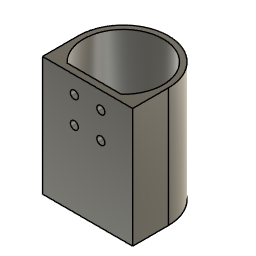
Tube v4 (Autodesk Fusion 360 design; units mm, degrees)
Autodesk Fusion 360 part; units mm, degrees
note: some values were not read from the file. Set by a fixed rule: which sketch regions a step uses.
sketch "Sketch1" plane through (0, 0, 0) normal (0, 0, 1) x (1, 0, 0)
  circle A0 centre (0, 0) radius 30
  circle A1 centre (0, 0) radius 34
  line L0 (0, 30) -> (0, -22) construction
  line L1 (-20.3961, -22) -> (20.3961, -22)
  line L2 (-34, -27) -> (34, -27)
  line L3 (-34, -27) -> (-34, 0)
  line L4 (34, -27) -> (34, 0)
  circle A2 centre (0, 4) radius 25.4 construction
  dimension "d1" = 60
  dimension "d2" = 68
  dimension "d3" = 52
  dimension "d6" = 5
  dimension "d38" = 50.8
  constraint coincident A0.centre A1.centre
  constraint coincident A0 L0.start
  constraint vertical L0
  constraint coincident A0.centre L0
  constraint coincident A0 L1.start
  constraint coincident A0 L1.end
  constraint horizontal L1
  constraint coincident L0.end L1
  constraint parallel L1 L2
  constraint coincident A1 L3.end
  constraint tangent A1 L3
  constraint coincident A1 L4.end
  constraint tangent A1 L4
  constraint vertical L4
  constraint vertical L3
  constraint midpoint L0 A2.centre
  measures "d1" diameter of A0
  measures "d2" diameter of A1
  measures "d3" distance of L0.start L0.end
  measures "d6" vertical distance of L1.start L2.start
  measures "d38" diameter of A2
extrude "Extrude1" add sketch "Sketch1" along normal blind 90 contours A0 A1 L2 | A0 L1 L2 | A1 L2 L3 | A1 L2 L4 picked at (-32.5234, 2.2674)
sketch "Sketch8" plane through (0, -27, 0) normal (0, -1, 0) x (1, 0, 0)
  line L0 (-34, 0) -> (34, 0)
  line L1 (34, 0) -> (34, 90)
  line L2 (34, 90) -> (-34, 90)
  line L3 (-34, 90) -> (-34, 0)
  circle A0 centre (-10, 77) radius 3.05
  circle A1 centre (10, 77) radius 3.05
  circle A2 centre (-10, 57) radius 3.05
  circle A3 centre (10, 57) radius 3.05
  dimension "d43" = 6.1
  dimension "d44" = 6.1
  dimension "d45" = 6.1
  dimension "d46" = 6.1
  dimension "d47" = 13
  dimension "d48" = 13
  dimension "d49" = 33
  dimension "d50" = 33
  dimension "d51" = 20
  dimension "d52" = 20
  dimension "d53" = 24
  dimension "d54" = 24
  measures "d43" diameter of A0
  measures "d44" diameter of A1
  measures "d45" diameter of A2
  measures "d46" diameter of A3
  measures "d47" distance of L2 A0.centre
  measures "d48" distance of L2 A1.centre
  measures "d49" distance of L2 A2.centre
  measures "d50" distance of L2 A3.centre
  measures "d51" distance of A0.centre A1.centre
  measures "d52" distance of A2.centre A3.centre
  measures "d53" distance of L1 A1.centre
  measures "d54" distance of L1 A3.centre
extrude "Extrude10" cut sketch "Sketch8" against normal blind 5 contours A0 | A1 | A2 | A3
equation "d44 = d43"
equation "d45 = d43"
equation "d46 = d43"
equation "d48 = d47"
equation "d50 = d49"
equation "d52 = d51"
equation "d54 = d53"
